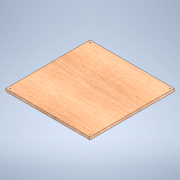
# Autodesk Inventor part: Base
Saved by Autodesk Inventor 2020 (Build 240168000, 168)
## iProperties
Created: 2020-03-15
Part Number: Base
Material: Wood (Birch)
Document SubType Name: Modeling
Designer: Peter
Density: 0.55 g/cm^3
Appearance: Birch - Natural Polished
Author: Peter
Autodesk Inventor part; units mm, degrees
ref_plane "YZ Plane" through (0, 0, 0) normal (1, 0, 0) x (0, 1, 0)
ref_plane "XZ Plane" through (0, 0, 0) normal (0, 1, 0) x (-1, 0, 0)
ref_plane "XY Plane" through (0, 0, 0) normal (0, 0, 1) x (1, 0, 0)
sketch "Sketch1" plane through (0, 0, 0) normal (0, 1, 0) x (-1, 0, 0)
  point P0 (0, 0)
sketch "Sketch2" plane through (0, 0, 0) normal (0, 1, 0) x (-1, 0, 0)
  line L0 (0, 0) -> (-400, 0)
  line L1 (-400, 0) -> (-400, -400)
  line L2 (-400, -400) -> (0, -400)
  line L3 (0, -400) -> (0, 0)
  dimension "d0" = 400
  dimension "d1" = 400
  constraints: 8 end point, 2 parallel, 1 horizontal, 1 perpendicular
  measures "d0" distance of L2.end L1.end
  measures "d1" distance of L1.end L0.end
extrude "Extrusion1" add sketch "Sketch2" along normal blind 12.7
sketch "Sketch3" plane through (0, 12.7, 0) normal (0, 1, 0) x (1, 0, 0)
  line L0 (400, 0) -> (400, 400) projected
  line L1 (400, 400) -> (0, 400) projected
  line L2 (0, 400) -> (0, 0) projected
  line L3 (0, 0) -> (400, 0) projected
  line L4 (10, 390) -> (390, 390)
  line L5 (390, 390) -> (390, 10)
  line L6 (390, 10) -> (10, 10)
  line L7 (10, 10) -> (10, 390)
  dimension "d4" = 10
  constraints: 8 end point, 3 other
  measures "d4" distance between parallel lines of L1 L4
hole "Hole1" at (10, 12.7, -390) at (10, 12.7, -10) at (390, 12.7, -390) at (390, 12.7, -10) direction (0, -1, 0) diameter 3.4 end through all clearance for "Countersunk Flat Head Screw DIN EN ISO 2009" size "M3" standard "DIN"
equation "\"d0\" = base_x_dim"
equation "\"d1\" = base_y_dim"
equation "\"d2\" = base_thickness"
equation "\"d4\" = 0.5 * extrusion_dim"
equation "\"base_y_dim\" = 400"
equation "\"base_x_dim\" = 400"
equation "\"base_thickness\" = 12.7"
equation "\"top_sheet_thickness\" = 6.35"
equation "\"extrusion_dim\" = 20"
body "Solid1"
